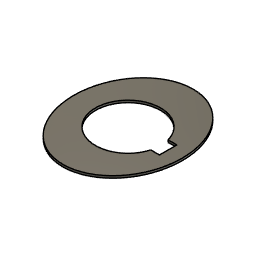
M365_stern_spacer (Autodesk Fusion 360 design; units mm, degrees)
Autodesk Fusion 360 part; units mm, degrees
sketch "Sketch1" plane through (0, 0, 0) normal (0, 1, 0) x (1, 0, 0)
  ellipse E0 centre (0, 0) end of major axis (0, 30) minor radius 25
  line L0 (0, -30) -> (0, 30) construction
  line L1 (25, 0) -> (-25, 0) construction
  circle A0 centre (0, 0) radius 15
  line L2 (0, 0) -> (18.5, 0)
  line L3 (18.5, 0) -> (18.5, 4)
  line L4 (18.5, 4) -> (14.4568, 4)
  line L5 (18.5, -4) -> (14.4568, -4)
  line L6 (18.5, 0) -> (18.5, -4)
  dimension "d1" = 60
  dimension "d2" = 50
  dimension "d3" = 30
  dimension "d4" = 18.5
  dimension "d5" = 4
  constraint coincident E0 L0.start
  constraint coincident E0 L0.end
  constraint coincident E0 L1.start
  constraint coincident E0 L1.end
  constraint coincident E0.centre A0.centre
  constraint vertical L0
  constraint coincident L1 L2.end
  constraint perpendicular L1 L3
  constraint coincident A0 L4.end
  constraint perpendicular L3 L4
  constraint symmetric L3.start L2 L6.start
  constraint symmetric L2 L3.end L5.start
  constraint symmetric L2 L4.end L5.end
  measures "d1" distance of E0
  measures "d3" diameter of A0
  measures "d4" distance of E0.centre L2.end
  measures "d5" distance of L2.end L3.end
extrude "Extrude1" add sketch "Sketch1" along normal blind 1
named bodies: "spacer"
